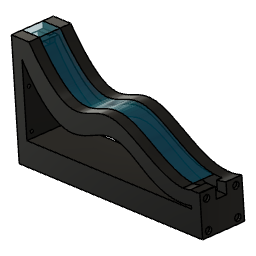
Light Fight Enclosure (Autodesk Fusion 360 archive; units mm, degrees)
design "curvy ramp v4"
Autodesk Fusion 360 part; units mm, degrees
sketch "Sketch1" plane through (0, 0, 0) normal (0, 0, 1) x (1, 0, 0)
  spline S0 degree 5 poles (40.6208, 29.6699) (42.6903, 29.0886) (46.8519, 28.1661) (53.162, 27.5032) (61.7121, 28.0705) (72.6192, 31.1607) (83.7085, 36.3916) (94.9004, 43.2126) (106.0422, 50.5427) (116.9303, 56.8759) (127.3997, 60.8059) (137.4036, 61.4785) (147.0888, 59.0274) (156.9108, 55.2199) (167.5566, 53.0755) (179.7979, 56.1158) (191.4539, 65.4249) (201.4947, 77.4532) (208.7977, 87.8654) (212.6014, 93.6699) knots 0 0 0 0 0 0 0.066667 0.133333 0.2 0.266667 0.333333 0.4 0.466667 0.533333 0.6 0.666667 0.733333 0.8 0.866667 0.933333 1 1 1 1 1 1
  line L0 (179.6654, 43.41) -> (245.5375, 143.9298)
  line L1 (220.9765, 77.3947) -> (220.9765, 14.5028)
  line L2 (220.9765, 14.5028) -> (50.4322, 14.5028)
  line L3 (40.6208, -6.3301) -> (230.6208, -6.3301)
  line L4 (230.6208, -6.3301) -> (230.6208, 93.6699)
  line L5 (230.6208, 93.6699) -> (220.6014, 93.6699)
  line L6 (212.6014, 93.6699) -> (220.6014, 93.6699)
  line L7 (40.6208, -6.3301) -> (40.6208, 29.6699)
  line L8 (50.4322, 25) -> (50.4322, 29.3521)
  line L9 (45.7339, 28.5315) -> (45.7339, 30.6355)
  spline S1 degree 5 poles (50.4322, 19.7514) (52.5083, 19.1803) (56.6446, 18.3262) (62.802, 17.9101) (70.9288, 19.0392) (81.0066, 22.914) (91.0633, 28.6513) (101.1387, 35.3847) (111.216, 41.8884) (121.2377, 46.7545) (131.1696, 48.8392) (141.0529, 47.6423) (151.0634, 43.7413) (161.5702, 39.235) (173.0579, 37.1534) (186.0507, 40.8953) (198.0377, 51.1113) (208.0884, 63.9296) (215.2808, 74.9049) (219, 81) knots 0 0 0 0 0 0 0.066667 0.133333 0.2 0.266667 0.333333 0.4 0.466667 0.533333 0.6 0.666667 0.733333 0.8 0.866667 0.933333 1 1 1 1 1 1
  line L10 (32.1869, 24.771) -> (68.6776, 14.7318)
  line L11 (195.2279, 42.0418) -> (242.7721, 119.9582)
  spline S2 degree 5 poles (50.4322, 16.9226) (52.4541, 16.5811) (56.4538, 16.0581) (62.3213, 15.7533) (69.8796, 16.3106) (78.8858, 18.5848) (87.4619, 22.3088) (95.6395, 27.1962) (103.481, 32.7303) (111.0878, 38.1115) (118.5811, 42.4666) (126.084, 45.0564) (133.7048, 45.46) (141.5155, 43.8368) (149.5479, 40.9254) (157.8081, 37.7616) (166.2852, 35.4807) (174.9619, 35.0844) (183.8239, 37.2317) (192.8597, 42.3178) (202.0608, 50.5416) (209.5491, 59.6845) (215.2356, 67.9818) (219.0577, 74.1509) (220.9765, 77.3947) knots 0 0 0 0 0 0 0.05 0.1 0.15 0.2 0.25 0.3 0.35 0.4 0.45 0.5 0.55 0.6 0.65 0.7 0.75 0.8 0.85 0.9 0.95 1 1 1 1 1 1
  line L12 (50.4322, 14.5028) -> (50.4322, 16.9226)
  line L13 (50.4322, 19.7514) -> (50.4322, 25)
  line L14 (214.982, 87.8743) -> (225.0015, 87.8743)
  line L15 (219, 87.8743) -> (219, 81)
  spline S3 degree 5 poles (45.7339, 30.6355) (46.5699, 30.3716) (48.2439, 29.874) (50.7614, 29.2181) (54.1786, 28.5327) (58.786, 28.0644) (63.9673, 28.117) (69.8324, 28.9007) (76.3745, 30.6358) (83.5069, 33.4676) (91.0889, 37.3911) (98.9572, 42.1572) (106.9497, 47.2251) (114.9161, 51.9215) (122.7278, 55.567) (130.2903, 57.6208) (137.5524, 57.8047) (144.5217, 56.274) (151.2654, 53.6563) (157.8841, 50.8259) (164.4905, 48.7284) (171.188, 48.2031) (178.0454, 49.7664) (185.0905, 53.5626) (192.324, 59.5003) (199.7286, 67.3358) (205.7693, 74.8869) (210.3553, 81.1578) (213.4359, 85.593) (214.982, 87.8743) knots 0 0 0 0 0 0 0.04 0.08 0.12 0.16 0.2 0.24 0.28 0.32 0.36 0.4 0.44 0.48 0.52 0.56 0.6 0.64 0.68 0.72 0.76 0.8 0.84 0.88 0.92 0.96 1 1 1 1 1 1
  line L16 (27.4957, 36.3931) -> (63.9722, 24.878)
  line L17 (199.1589, 64.5274) -> (230.8052, 111.2212)
  line L18 (225.0015, 93.6699) -> (225.0015, 87.8743)
  line L19 (219, 81) -> (230.6208, 81)
  line L20 (50.4322, 29.3521) -> (40.6208, 29.3521)
  line L21 (50.4322, 19.7514) -> (40.6208, 19.7514)
  line L22 (225.0015, 87.8743) -> (230.6208, 87.8743)
  point P0 (90.0597, 40.3798)
  point P1 (140.0597, 60.3798)
  point P2 (169.2008, 69.6255)
  point P3 (141, 47)
  point P4 (96, 32)
  point P5 (59.7278, 28.1711)
  point P6 (89.6315, 36.7573)
  point P7 (135.0748, 57.5007)
  point P8 (167.951, 48.6886)
  point P9 (95, 27)
  point P10 (130, 45)
  point P11 (166, 36)
  dimension "d1" = 36
  dimension "d2" = 8
  dimension "d3" = 190
  dimension "d63" = 100
  constraint vertical L7
  constraint horizontal L6
  constraint perpendicular L3 L7
  constraint perpendicular L3 L4
  constraint perpendicular L4 L5
  constraint perpendicular L1 L5
  constraint perpendicular L1 L2
  constraint perpendicular L2 L12
  constraint midpoint S0.end L0
  constraint parallel L8 L12
  constraint coincident S0 L9.start
  constraint vertical L9
  constraint coincident L8.end S3
  constraint coincident S1.start L12
  constraint midpoint S1.start L10
  constraint midpoint S1.end L11
  constraint collinear L12 L13
  constraint perpendicular L4 L14
  constraint coincident L14 L15.start
  constraint midpoint L9.end L16
  constraint midpoint L14.start L17
  constraint coincident L5 L18.start
  constraint perpendicular L14 L18
  constraint coincident L4 L19.end
  constraint perpendicular L4 L19
  constraint coincident L7 L20.end
  constraint perpendicular L7 L20
  constraint coincident L7 L21.end
  constraint coincident L4 L22.end
  constraint perpendicular L4 L22
  measures "d1" distance of L3.start S0.start
  measures "d2" distance of S0.end L5.end
  measures "d3" distance of L3.start L3.end
  measures "d63" distance of L3.end L4.end
extrude "Extrude5" add sketch "Sketch1" along normal blind 40 contours S0 L7 L20 | S0 L7 L8 L10 L13 L20 | L7 L10 L21 | S0 L8 S1 L13 L14 L15 S3 | L1 L2 L3 L4 L7 L10 L11 S2 L12 L19 L21 | S1 L10 L11 S2 | L11 L14 L15 | L4 L11 L14 L19 L22 | S0 L0 S3 | L5 L6 L11 L14 L17 L18 | L11 L14 L18 | L0 L6 S3 L17 | L5 L11 L18 | L4 L5 L11 L18 L22 makes body 1
extrude "Extrude6" cut sketch "Sketch1" along normal blind 30 contours S0 L8 L16 | S0 L8 S1 L13 L14 L15 S3 | S0 L8 S3 L16 | S0 L0 S3 | L5 L6 L11 L14 L17 L18 | L11 L14 L18 | L0 L6 S3 L17 bodies 1
extrude "Extrude7" cut sketch "Sketch1" along normal blind 25 contours S0 L7 L20 | S0 L9 L20 | S0 L7 L8 L10 L13 L20 | S0 L8 L9 L16 L20 | L7 L10 L21 | L8 L16 L20 | L11 L14 L15 | L4 L11 L14 L19 L22 | L5 L11 L18 | L4 L5 L11 L18 L22 bodies 1
extrude "Extrude8" add sketch "Sketch1" along normal blind 15 contours S0 L7 L20 | S0 L9 L20 | S0 L7 L8 L10 L13 L20 | S0 L8 L9 L16 L20 | L7 L10 L21 | L8 L16 L20 | L11 L14 L15 | L4 L11 L14 L19 L22 | L5 L11 L18 | L4 L5 L11 L18 L22 bodies 1
extrude "Extrude9" add sketch "Sketch1" along normal blind 10 contours S0 L8 L16 | S0 L8 S1 L13 L14 L15 S3 | S0 L8 S3 L16 | S0 L0 S3 | L5 L6 L11 L14 L17 L18 | L11 L14 L18 | L0 L6 S3 L17 bodies 1
extrude "Extrude11" cut sketch "Sketch1" along normal blind 30 contours L5 L11 L18 | L4 L5 L11 L18 L22 bodies 1
extrude "Extrude12" add sketch "Sketch1" along normal blind 10 contours L5 L11 L18 | L4 L5 L11 L18 L22 bodies 1
extrude "Extrude13" add sketch "Sketch1" along normal blind 20 separate body contours S0 L0 S3 | L5 L6 L11 L14 L17 L18 | L11 L14 L18 | L0 L6 S3 L17 | L5 L11 L18 | L4 L5 L11 L18 L22 makes body 2
move_body "Move6" bodies 2 to x (1, 0, 0) y (0, 1, 0) z (0, 0, 1) at (0, 0, 10)
sketch "Sketch2" plane through (40.6208, 0, 0) normal (-1, 0, 0) x (0, -1, 0)
  line L0 (-29.6699, 25) -> (-19.7514, 25)
  line L1 (-19.7514, 25) -> (-19.7514, 15)
  line L2 (-19.7514, 15) -> (-29.6699, 15)
  line L3 (-29.6699, 15) -> (-29.6699, 0)
  line L4 (-29.6699, 0) -> (6.3301, 0)
  line L5 (6.3301, 0) -> (6.3301, 40)
  line L6 (6.3301, 40) -> (-29.6699, 40)
  line L7 (-29.6699, 40) -> (-29.6699, 25)
  circle A0 centre (-23.6699, 6) radius 2.95
  circle A1 centre (-23.6699, 34) radius 2.95
  circle A2 centre (1.3301, 6) radius 2.95
  circle A3 centre (1.3301, 34) radius 2.95
  dimension "d34" = 5.9
  dimension "d35" = 5.9
  dimension "d36" = 5.9
  dimension "d37" = 5.9
  dimension "d65" = 6
  dimension "d66" = 6
  dimension "d67" = 6
  dimension "d68" = 25
  dimension "d69" = 6
  dimension "d70" = 6
  dimension "d71" = 25
  dimension "d72" = 6
  measures "d34" diameter of A0
  measures "d35" diameter of A1
  measures "d36" diameter of A2
  measures "d37" diameter of A3
  measures "d65" distance of L7 A1.centre
  measures "d66" distance of L6 A1.centre
  measures "d67" distance of L6 A3.centre
  measures "d68" distance of A1.centre A3.centre
  measures "d69" distance of L3 A0.centre
  measures "d70" distance of L4 A0.centre
  measures "d71" horizontal distance of A0.centre A2.centre
  measures "d72" distance of L4 A2.centre
extrude "Extrude14" cut sketch "Sketch2" against normal blind 2.4 contours A0 | A1 | A2 | A3 bodies 1
sketch "Sketch3" plane through (230.6208, 0, 0) normal (1, 0, 0) x (0, 1, 0)
  line L0 (87.8743, 10) -> (87.8743, 15)
  line L1 (87.8743, 15) -> (81, 15)
  line L2 (81, 15) -> (81, 25)
  line L3 (81, 25) -> (87.8743, 25)
  line L4 (87.8743, 25) -> (87.8743, 30)
  line L5 (87.8743, 30) -> (93.6699, 30)
  line L6 (93.6699, 30) -> (93.6699, 40)
  line L7 (93.6699, 40) -> (-6.3301, 40)
  line L8 (-6.3301, 40) -> (-6.3301, 0)
  line L9 (-6.3301, 0) -> (93.6699, 0)
  line L10 (93.6699, 0) -> (93.6699, 10)
  line L11 (93.6699, 10) -> (87.8743, 10)
  circle A0 centre (55, 35) radius 2.95
  circle A1 centre (55, 35) radius 2.95
  circle A2 centre (55, 35) radius 1.5
  circle A3 centre (55, 35) radius 1.5
  circle A4 centre (55, 5) radius 2.95
  circle A5 centre (55, 5) radius 2.95
  circle A6 centre (55, 5) radius 1.5
  circle A7 centre (55, 5) radius 1.5
  circle A8 centre (20, 35) radius 2.95
  circle A9 centre (20, 35) radius 2.95
  circle A10 centre (20, 35) radius 1.5
  circle A11 centre (20, 35) radius 1.5
  circle A12 centre (20, 5) radius 1.5
  circle A13 centre (20, 5) radius 1.5
  circle A14 centre (20, 5) radius 2.95
  circle A15 centre (20, 5) radius 2.95
  point P0 (55, 35)
  point P1 (55, 35)
  point P2 (55, 5)
  point P3 (55, 5)
  point P4 (20, 35)
  point P5 (20, 35)
  point P6 (20, 5)
  point P7 (20, 5)
  dimension "d40" = 5.9
  dimension "d41" = 5.9
  dimension "d45" = 3
  dimension "d46" = 3
  dimension "d47" = 5.9
  dimension "d48" = 5.9
  dimension "d49" = 3
  dimension "d50" = 3
  dimension "d51" = 5.9
  dimension "d52" = 5.9
  dimension "d53" = 3
  dimension "d54" = 3
  dimension "d55" = 5.9
  dimension "d56" = 5.9
  dimension "d57" = 3
  dimension "d58" = 3
  constraint concentric A0 A2
  constraint concentric A4 A6
  constraint concentric A8 A10
  constraint concentric A12 A14
  measures "d40" diameter of A0
  measures "d41" diameter of A1
  measures "d45" diameter of A2
  measures "d46" diameter of A3
  measures "d47" diameter of A4
  measures "d48" diameter of A5
  measures "d49" diameter of A6
  measures "d50" diameter of A7
  measures "d51" diameter of A8
  measures "d52" diameter of A9
  measures "d53" diameter of A10
  measures "d54" diameter of A11
  measures "d55" diameter of A14
  measures "d56" diameter of A15
  measures "d57" diameter of A12
  measures "d58" diameter of A13
extrude "Extrude15" cut sketch "Sketch3" against normal blind 2.4 contours A0 A1 | A2 A3 | A4 A5 | A6 A7 | A8 A9 | A10 A11 | A12 A13 | A14 A15 bodies 1
extrude "Extrude16" cut sketch "Sketch3" against normal blind 10 contours A2 A3 | A6 A7 | A10 A11 | A12 A13 bodies 1
equation "neopixelwidth = 20 mm"
equation "sidethickness = 10 mm"
equation "d30 = neopixelwidth"
equation "magneddiam = 5.9 mm"
equation "magnetDepth = 2.4 mm"
equation "d34 = magneddiam"
equation "d35 = magneddiam"
equation "d36 = magneddiam"
equation "d37 = magneddiam"
equation "d38 = -magnetDepth"
equation "d40 = magneddiam"
equation "d41 = magneddiam"
equation "d47 = magneddiam"
equation "d48 = magneddiam"
equation "d51 = magneddiam"
equation "d52 = magneddiam"
equation "d55 = magneddiam"
equation "d56 = magneddiam"
equation "d59 = -magnetDepth"
named bodies: "blackPLA", "clearPLA"
